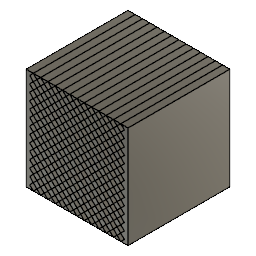
Crosshatch v1 (Autodesk Fusion 360 design; units mm, degrees)
Autodesk Fusion 360 part; units mm, degrees
sketch "Sketch1" plane through (0, 0, 0) normal (0, 1, 0) x (1, 0, 0)
  line L0 (0, -25) -> (70, -25)
  line L1 (70, -25) -> (70, 45)
  line L2 (70, 45) -> (0, 45)
  line L3 (0, 45) -> (0, -25)
  line L4 (0, 40) -> (5, 45)
  line L5 (0, 35) -> (10, 45)
  line L6 (0, 30) -> (15, 45)
  line L7 (0, 25) -> (20, 45)
  line L8 (0, 20) -> (25, 45)
  line L9 (0, 15) -> (30, 45)
  line L10 (0, 10) -> (35, 45)
  line L11 (0, 5) -> (40, 45)
  line L12 (0, 0) -> (45, 45)
  line L13 (0, -5) -> (50, 45)
  line L14 (0, -10) -> (55, 45)
  line L15 (0, -15) -> (60, 45)
  line L16 (0, -20) -> (65, 45)
  line L17 (0, -25) -> (70, 45)
  line L18 (65, -25) -> (70, -20)
  line L19 (60, -25) -> (70, -15)
  line L20 (55, -25) -> (70, -10)
  line L21 (50, -25) -> (70, -5)
  line L22 (45, -25) -> (70, 0)
  line L23 (40, -25) -> (70, 5)
  line L24 (35, -25) -> (70, 10)
  line L25 (30, -25) -> (70, 15)
  line L26 (25, -25) -> (70, 20)
  line L27 (20, -25) -> (70, 25)
  line L28 (15, -25) -> (70, 30)
  line L29 (10, -25) -> (70, 35)
  line L30 (5, -25) -> (70, 40)
  line L31 (0, -20) -> (5, -25)
  line L32 (0, -15) -> (10, -25)
  line L33 (0, -10) -> (15, -25)
  line L34 (0, -5) -> (20, -25)
  line L35 (0, 0) -> (25, -25)
  line L36 (0, 5) -> (30, -25)
  line L37 (0, 10) -> (35, -25)
  line L38 (0, 15) -> (40, -25)
  line L39 (0, 20) -> (45, -25)
  line L40 (0, 25) -> (50, -25)
  line L41 (0, 30) -> (55, -25)
  line L42 (0, 35) -> (60, -25)
  line L43 (0, 40) -> (65, -25)
  line L44 (0, 45) -> (70, -25)
  line L45 (5, 45) -> (70, -20)
  line L46 (10, 45) -> (70, -15)
  line L47 (15, 45) -> (70, -10)
  line L48 (20, 45) -> (70, -5)
  line L49 (25, 45) -> (70, 0)
  line L50 (30, 45) -> (70, 5)
  line L51 (35, 45) -> (70, 10)
  line L52 (40, 45) -> (70, 15)
  line L53 (45, 45) -> (70, 20)
  line L54 (50, 45) -> (70, 25)
  line L55 (55, 45) -> (70, 30)
  line L56 (60, 45) -> (70, 35)
  line L57 (65, 45) -> (70, 40)
  dimension "d1" = 70
  dimension "d2" = 70
extrude "Extrude1" add sketch "Sketch1" along normal blind 70 contours L0 L17 L31 | L3 L17 L31 | L0 L30 L32 | L3 L16 L32 | L16 L17 L31 L32 | L0 L29 L33 | L17 L30 L32 L33 | L3 L15 L33 | L15 L16 L32 L33 | L0 L28 L34 | L29 L30 L33 L34 | L3 L14 L34 | L14 L15 L33 L34 | L16 L17 L33 L34 | L0 L27 L35 | L28 L29 L34 L35 | L17 L30 L34 L35 | L3 L13 L35 | L13 L14 L34 L35 | L15 L16 L34 L35 | L0 L26 L36 | L27 L28 L35 L36 | L29 L30 L35 L36 | L3 L12 L36 | L12 L13 L35 L36 | L14 L15 L35 L36 | L16 L17 L35 L36 | L0 L25 L37 | L26 L27 L36 L37 | L28 L29 L36 L37 | L17 L30 L36 L37 | L3 L11 L37 | L11 L12 L36 L37 | L13 L14 L36 L37 | L15 L16 L36 L37 | L0 L24 L38 | L25 L26 L37 L38 | L27 L28 L37 L38 | L29 L30 L37 L38 | L3 L10 L38 | L10 L11 L37 L38 | L12 L13 L37 L38 | L14 L15 L37 L38 | L16 L17 L37 L38 | L0 L23 L39 | L24 L25 L38 L39 | L26 L27 L38 L39 | L28 L29 L38 L39 | L17 L30 L38 L39 | L3 L9 L39 | L9 L10 L38 L39 | L11 L12 L38 L39 | L13 L14 L38 L39 | L15 L16 L38 L39 | L0 L22 L40 | L23 L24 L39 L40 | L25 L26 L39 L40 | L27 L28 L39 L40 | L29 L30 L39 L40 | L3 L8 L40 | L8 L9 L39 L40 | L10 L11 L39 L40 | L12 L13 L39 L40 | L14 L15 L39 L40 | L16 L17 L39 L40 | L0 L21 L41 | L22 L23 L40 L41 | L24 L25 L40 L41 | L26 L27 L40 L41 | L28 L29 L40 L41 | L17 L30 L40 L41 | L3 L7 L41 | L7 L8 L40 L41 | L9 L10 L40 L41 | L11 L12 L40 L41 | L13 L14 L40 L41 | L15 L16 L40 L41 | L0 L20 L42 | L21 L22 L41 L42 | L23 L24 L41 L42 | L25 L26 L41 L42 | L27 L28 L41 L42 | L29 L30 L41 L42 | L3 L6 L42 | L6 L7 L41 L42 | L8 L9 L41 L42 | L10 L11 L41 L42 | L12 L13 L41 L42 | L14 L15 L41 L42 | L16 L17 L41 L42 | L0 L19 L43 | L20 L21 L42 L43 | L22 L23 L42 L43 | L24 L25 L42 L43 | L26 L27 L42 L43 | L28 L29 L42 L43 | L17 L30 L42 L43 | L3 L5 L43 | L5 L6 L42 L43 | L7 L8 L42 L43 | L9 L10 L42 L43 | L11 L12 L42 L43 | L13 L14 L42 L43 | L15 L16 L42 L43 | L0 L18 L44 | L19 L20 L43 L44 | L21 L22 L43 L44 | L23 L24 L43 L44 | L25 L26 L43 L44 | L27 L28 L43 L44 | L29 L30 L43 L44 | L3 L4 L44 | L4 L5 L43 L44 | L6 L7 L43 L44 | L8 L9 L43 L44 | L10 L11 L43 L44 | L12 L13 L43 L44 | L14 L15 L43 L44 | L16 L17 L43 L44 | L1 L18 L44 | L18 L19 L44 L45 | L20 L21 L44 L45 | L22 L23 L44 L45 | L24 L25 L44 L45 | L26 L27 L44 L45 | L28 L29 L44 L45 | L17 L30 L44 L45 | L2 L4 L44 | L5 L6 L44 L45 | L7 L8 L44 L45 | L9 L10 L44 L45 | L11 L12 L44 L45 | L13 L14 L44 L45 | L15 L16 L44 L45 | L1 L19 L45 | L19 L20 L45 L46 | L21 L22 L45 L46 | L23 L24 L45 L46 | L25 L26 L45 L46 | L27 L28 L45 L46 | L29 L30 L45 L46 | L2 L5 L45 | L6 L7 L45 L46 | L8 L9 L45 L46 | L10 L11 L45 L46 | L12 L13 L45 L46 | L14 L15 L45 L46 | L16 L17 L45 L46 | L1 L20 L46 | L20 L21 L46 L47 | L22 L23 L46 L47 | L24 L25 L46 L47 | L26 L27 L46 L47 | L28 L29 L46 L47 | L17 L30 L46 L47 | L2 L6 L46 | L7 L8 L46 L47 | L9 L10 L46 L47 | L11 L12 L46 L47 | L13 L14 L46 L47 | L15 L16 L46 L47 | L1 L21 L47 | L21 L22 L47 L48 | L23 L24 L47 L48 | L25 L26 L47 L48 | L27 L28 L47 L48 | L29 L30 L47 L48 | L2 L7 L47 | L8 L9 L47 L48 | L10 L11 L47 L48 | L12 L13 L47 L48 | L14 L15 L47 L48 | L16 L17 L47 L48 | L1 L22 L48 | L22 L23 L48 L49 | L24 L25 L48 L49 | L26 L27 L48 L49 | L28 L29 L48 L49 | L17 L30 L48 L49 | L2 L8 L48 | L9 L10 L48 L49 | L11 L12 L48 L49 | L13 L14 L48 L49 | L15 L16 L48 L49 | L1 L23 L49 | L23 L24 L49 L50 | L25 L26 L49 L50 | L27 L28 L49 L50 | L29 L30 L49 L50 | L2 L9 L49 | L10 L11 L49 L50 | L12 L13 L49 L50 | L14 L15 L49 L50 | L16 L17 L49 L50 | L1 L24 L50 | L24 L25 L50 L51 | L26 L27 L50 L51 | L28 L29 L50 L51 | L17 L30 L50 L51 | L2 L10 L50 | L11 L12 L50 L51 | L13 L14 L50 L51 | L15 L16 L50 L51 | L1 L25 L51 | L25 L26 L51 L52 | L27 L28 L51 L52 | L29 L30 L51 L52 | L2 L11 L51 | L12 L13 L51 L52 | L14 L15 L51 L52 | L16 L17 L51 L52 | L1 L26 L52 | L26 L27 L52 L53 | L28 L29 L52 L53 | L17 L30 L52 L53 | L2 L12 L52 | L13 L14 L52 L53 | L15 L16 L52 L53 | L1 L27 L53 | L27 L28 L53 L54 | L29 L30 L53 L54 | L2 L13 L53 | L14 L15 L53 L54 | L16 L17 L53 L54 | L1 L28 L54 | L28 L29 L54 L55 | L17 L30 L54 L55 | L2 L14 L54 | L15 L16 L54 L55 | L1 L29 L55 | L29 L30 L55 L56 | L2 L15 L55 | L16 L17 L55 L56 | L1 L30 L56 | L17 L30 L56 L57 | L2 L16 L56 | L1 L17 L57 | L2 L17 L57
